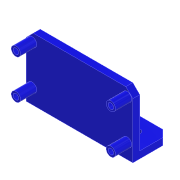
# Autodesk Inventor part: ultrasonic mount (front) v2
Saved by Autodesk Inventor 2022 (Build 260153000, 153)
## iProperties
Created: 2024-06-19
Part Number: ultrasonic mount (front) v2
Material: Generic
Document SubType Name: Modeling
Designer: david
Density: 1 g/cm^3
Appearance: Smooth - Dark Forest Green
Author: david
Autodesk Inventor part; units mm, degrees
ref_plane "YZ Plane" through (0, 0, 0) normal (1, 0, 0) x (0, 1, 0)
ref_plane "XZ Plane" through (0, 0, 0) normal (0, 1, 0) x (-1, 0, 0)
ref_plane "XY Plane" through (0, 0, 0) normal (0, 0, 1) x (1, 0, 0)
sketch "Sketch1" plane through (0, 0, 0) normal (0, 0, 1) x (1, 0, 0)
  line L0 (-22, 22) -> (22, 22) construction
  line L1 (22, 22) -> (22, 2) construction
  line L2 (22, 2) -> (-22, 2) construction
  line L3 (-22, 2) -> (-22, 22) construction
  line L4 (-22, 22) -> (22, 2) construction
  line L5 (22, 22) -> (-22, 2) construction
  line L6 (23, 24) -> (-23, 24)
  line L7 (-23, 24) -> (-23, 0)
  line L8 (-23, 0) -> (23, 0)
  line L9 (23, 0) -> (23, 24)
  point P0 (0, 12)
  point P1 (0, 12)
  point P2 (0, 0)
  point P3 (0, 12)
  dimension "d0" = 20
  dimension "d1" = 44
  dimension "d2" = 2
  dimension "d60" = 2
  dimension "d61" = 1
  dimension "d62" = 1
  constraints: 20 end point, 5 midpoint, 4 parallel, 2 perpendicular, 1 horizontal, 1 vertical alignment
  measures "d0" distance of L0.end L1.end
  measures "d1" distance of L1.end L2.end
  measures "d2" distance between parallel lines of L0 L6
  measures "d60" distance between parallel lines of L8 L2
  measures "d61" distance between parallel lines of L9 L1
  measures "d62" distance between parallel lines of L7 L3
extrude "Extrusion1" add sketch "Sketch1" against normal blind 3
sketch "Sketch2" plane through (-23, 0, 0) normal (0, -1, 0) x (1, 0, 0)
  line L0 (0, 0) -> (46, 0)
  line L1 (46, 0) -> (46, -16)
  line L2 (46, -16) -> (0, -16)
  line L3 (0, -16) -> (0, 0)
  line L4 (46, 0) -> (0, 0) projected
  line L5 (46, 0) -> (46, -3) projected
  line L6 (0, 0) -> (0, -3) projected
  point P0 (23, 0)
  dimension "d54" = 46
  dimension "d55" = 16
  dimension "d59" = 46
  constraints: 8 end point, 2 midpoint, 2 parallel, 1 collinear, 1 horizontal, 1 perpendicular
  measures "d54" distance of L1.end L2.end
  measures "d55" distance of L0.end L1.end
  measures "d59" distance between parallel lines of L5 L6
extrude "Extrusion2" add sketch "Sketch2" along normal blind 3
sketch "Sketch3" plane through (0, 0, 0) normal (0, 0, 1) x (1, 0, 0)
  line L0 (-21.5, 21.5) -> (21.5, 21.5) construction
  line L1 (21.5, 21.5) -> (21.5, 2.5) construction
  line L2 (21.5, 2.5) -> (-21.5, 2.5) construction
  line L3 (-21.5, 2.5) -> (-21.5, 21.5) construction
  circle A0 centre (-20.5, 20.5) radius 1 construction
  circle A1 centre (-20.5, 3.5) radius 1 construction
  circle A2 centre (20.5, 20.5) radius 1 construction
  circle A3 centre (20.5, 3.5) radius 1 construction
  line L4 (23, 24) -> (23, 0) projected
  line L5 (22, 22) -> (-22, 22)
  line L6 (-22, 22) -> (-22, 2)
  line L7 (-22, 2) -> (22, 2)
  line L8 (22, 2) -> (22, 22)
  point P0 (0, 0)
  point P1 (0, 2.5)
  point P2 (21.5, 12)
  point P3 (23, 12)
  point P4 (23, 0)
  point P5 (24, 3)
  dimension "d8" = 2
  dimension "d9" = 2
  dimension "d10" = 2
  dimension "d11" = 2
  dimension "d43" = 0.5
  dimension "d44" = 44
  dimension "d45" = 20
  constraints: 16 end point, 8 tangent, 4 centre point, 4 coincident, 4 parallel, 2 midpoint, 2 perpendicular, 1 horizontal, 1 horizontal alignment, 1 vertical alignment, 5 other
  measures "d8" diameter of A0
  measures "d9" diameter of A2
  measures "d10" diameter of A3
  measures "d11" diameter of A1
  measures "d43" distance between parallel lines of L5 L0
  measures "d44" distance between parallel lines of L6 L8
  measures "d45" distance of L5.end L6.end
hole "Hole1" at (-20.5, 20.5, 0) at (20.5, 20.5, 0) at (20.5, 3.5, 0) at (-20.5, 3.5, 0) direction (0, 0, -1) diameter 2.4 depth 6
sketch "Sketch5" plane through (-23, 0, 0) normal (0, 1, 0) x (1, 0, 0)
  line L0 (0, 3) -> (46, 3) projected
  line L1 (46, 0) -> (0, 0) projected
  line L2 (46, 16) -> (46, 3) projected
  line L3 (0, 3) -> (0, 16) projected
  line L4 (0, 16) -> (46, 16) projected
  line L5 (46, 16) -> (46, 3) projected
  line L6 (0, 3) -> (46, 3) projected
  line L7 (0, 3) -> (0, 16) projected
  line L8 (0, 16) -> (46, 16) projected
  line L9 (46, 0) -> (0, 0) projected
  line L10 (8, 9.5) -> (38, 9.5)
  line L11 (0, 0) -> (0, 3) projected
  line L12 (46, 3) -> (46, 0) projected
  line L13 (0, 0) -> (0, 3) projected
  line L14 (46, 3) -> (46, 0) projected
  point P0 (23, 9.5)
  point P1 (23, 16)
  dimension "d56" = 13
  dimension "d57" = 6.5
  dimension "d58" = 30
  constraints: 2 end point, 2 midpoint, 1 horizontal, 1 vertical alignment
  measures "d56" distance between parallel lines of L4 L0
  measures "d57" distance between parallel lines of L4 L10
  measures "d58" distance of L10.end L10.start
hole "Hole2" at (-15, 0, -9.5) at (15, 0, -9.5) direction (0, -1, 0) diameter 3.4 depth 6
chamfer "Chamfer2" distance 3 angle 45 4 edges at (-23, 24, -1.5) (23, 24, -1.5) (23, -1.5, -16) (-23, -1.5, -16)
sketch "Sketch6" plane through (0, 0, 0) normal (0, 0, 1) x (1, 0, 0)
  circle A0 centre (-20.5, 20.5) radius 1.2 projected
  circle A1 centre (-20.5, 20.5) radius 2
  circle A2 centre (20.5, 20.5) radius 1.2 projected
  circle A3 centre (20.5, 20.5) radius 2
  circle A4 centre (20.5, 3.5) radius 1.2 projected
  circle A5 centre (20.5, 3.5) radius 2
  circle A6 centre (-20.5, 3.5) radius 1.2 projected
  circle A7 centre (-20.5, 3.5) radius 2
  point P0 (0, 0)
  dimension "d46" = 4
  dimension "d47" = 4
  dimension "d49" = 4
  dimension "d50" = 4
  constraints: 4 centre point, 4 coincident
  measures "d46" diameter of A1
  measures "d47" diameter of A3
  measures "d49" diameter of A5
  measures "d50" diameter of A7
extrude "Extrusion3" add sketch "Sketch6" along normal blind 7
equation "\"d60\" = d2"
equation "\"d62\" = d61"
equation "\"d54\" = d59"
equation "\"d44\" = d1"
equation "\"d45\" = d0"
equation "\"d57\" = 0.5 * d56"
equation "\"d46\" = d50"
equation "\"d47\" = d50"
equation "\"d49\" = d50"
body "Solid1"
